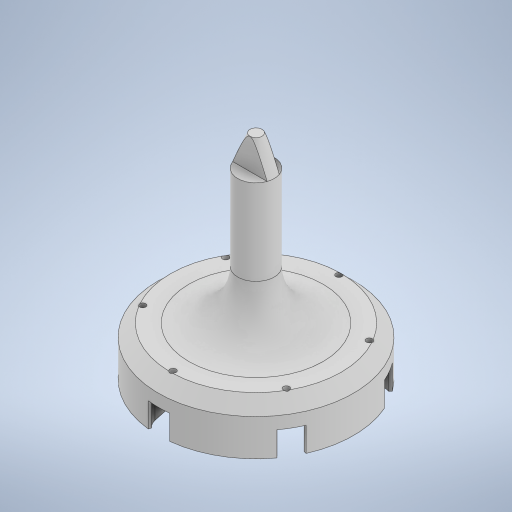
# Autodesk Inventor part: End_Effecto_simpler
Saved by Autodesk Inventor 2023 (Build 270158000, 158)
## iProperties
Created: 2025-02-16
Part Number: End_Effecto_simpler
Material: Generic
Document SubType Name: Modeling
Designer: Swoby
Density: 1 g/cm^3
Appearance: Default
Author: Swoby
Autodesk Inventor part; units mm, degrees
ref_plane "YZ Plane" through (0, 0, 0) normal (1, 0, 0) x (0, 1, 0)
ref_plane "XZ Plane" through (0, 0, 0) normal (0, 1, 0) x (-1, 0, 0)
ref_plane "XY Plane" through (0, 0, 0) normal (0, 0, 1) x (1, 0, 0)
sketch "Sketch1" plane through (0, 0, 0) normal (0, 0, 1) x (1, 0, 0)
  line L0 (0, 0) -> (0, 35)
  line L1 (0, 0) -> (-16, 0)
  line L2 (-16, 0) -> (-16, 8)
  line L3 (-3, 30) -> (0, 30) construction
  line L4 (-3, 30) -> (-3, 16)
  line L5 (-16, 8) -> (-11, 8)
  arc A0 (-11, 8) -> (-3, 16) centre (-11, 16) ccw
  line L6 (0, 35) -> (-1, 35)
  line L7 (-1, 35) -> (-3, 30)
  dimension "d0" = 32
  dimension "d1" = 30
  dimension "d2" = 6
  dimension "d4" = 8
  dimension "d7" = 8
  dimension "d8" = 5
  dimension "d10" = 1
  dimension "d34" = 8
  constraints: 16 end point, 3 horizontal, 2 point on circle, 2 vertical, 1 centre point, 1 parallel, 1 perpendicular, 1 point on line, 1 tangent
  measures "d0" diameter of L2 L0
  measures "d1" distance between parallel lines of L1 L3
  measures "d2" diameter of L3.start L0
  measures "d4" distance of L1.end L2.end
  measures "d7" distance from line of L5.end L4
  measures "d8" vertical distance of L3.start L0.end
  measures "d10" distance of L0.end L6.end
  measures "d34" distance from line of L4.end L5
revolve "Revolution1" add sketch "Sketch1" angle 360 about axis through (0, 0, 0) along (0, 1, 0)
chamfer "Chamfer1" distance 2 angle 45 1 edges at (16, 8, 0)
sketch "Sketch2" plane through (0, 0, 0) normal (0, -1, 0) x (1, 0, 0)
  arc A0 (-2.4436, -14.1282) -> (0, -16.1) centre (0, -13.6) ccw
  arc A1 (-13.943, -8.05) -> (-11.0136, -9.1803) centre (-11.7779, -6.8) ccw
  line L0 (0, -16.1) -> (0, 0) construction
  line L1 (0, 0) -> (-13.943, -8.05) construction
  circle A2 centre (0, 0) radius 8 construction
  line L2 (0, 0) -> (-4, -6.9282) construction
  line L3 (-3.9534, -7.1438) -> (-2.4436, -14.1282)
  line L4 (-4.21, -6.9956) -> (-11.0136, -9.1803)
  arc A3 (-3.9534, -7.1438) -> (-4.21, -6.9956) centre (-4.1489, -7.1861) ccw
  circle A4 centre (0, -13.6) radius 0.5
  circle A5 centre (11.7779, -6.8) radius 0.5
  arc A6 (11.0136, -9.1803) -> (13.943, -8.05) centre (11.7779, -6.8) ccw
  line L5 (4.21, -6.9956) -> (11.0136, -9.1803)
  arc A7 (4.21, -6.9956) -> (3.9534, -7.1438) centre (4.1489, -7.1861) ccw
  line L6 (3.9534, -7.1438) -> (2.4436, -14.1282)
  arc A8 (0, -16.1) -> (2.4436, -14.1282) centre (0, -13.6) ccw
  circle A9 centre (11.7779, 6.8) radius 0.5
  arc A10 (13.4572, 4.9479) -> (13.943, 8.05) centre (11.7779, 6.8) ccw
  line L7 (8.1634, 0.1482) -> (13.4572, 4.9479)
  arc A11 (8.1634, 0.1482) -> (8.1634, -0.1482) centre (8.2978, 0) ccw
  line L8 (8.1634, -0.1482) -> (13.4572, -4.9479)
  arc A12 (13.943, -8.05) -> (13.4572, -4.9479) centre (11.7779, -6.8) ccw
  circle A13 centre (0, 13.6) radius 0.5
  arc A14 (2.4436, 14.1282) -> (0, 16.1) centre (0, 13.6) ccw
  line L9 (3.9534, 7.1438) -> (2.4436, 14.1282)
  arc A15 (3.9534, 7.1438) -> (4.21, 6.9956) centre (4.1489, 7.1861) ccw
  line L10 (4.21, 6.9956) -> (11.0136, 9.1803)
  arc A16 (13.943, 8.05) -> (11.0136, 9.1803) centre (11.7779, 6.8) ccw
  circle A17 centre (-11.7779, 6.8) radius 0.5
  arc A18 (-11.0136, 9.1803) -> (-13.943, 8.05) centre (-11.7779, 6.8) ccw
  line L11 (-4.21, 6.9956) -> (-11.0136, 9.1803)
  arc A19 (-4.21, 6.9956) -> (-3.9534, 7.1438) centre (-4.1489, 7.1861) ccw
  line L12 (-3.9534, 7.1438) -> (-2.4436, 14.1282)
  arc A20 (0, 16.1) -> (-2.4436, 14.1282) centre (0, 13.6) ccw
  circle A21 centre (-11.7779, -6.8) radius 0.5
  arc A22 (-13.4572, -4.9479) -> (-13.943, -8.05) centre (-11.7779, -6.8) ccw
  line L13 (-8.1634, -0.1482) -> (-13.4572, -4.9479)
  arc A23 (-8.1634, -0.1482) -> (-8.1634, 0.1482) centre (-8.2978, 0) ccw
  line L14 (-8.1634, 0.1482) -> (-13.4572, 4.9479)
  arc A24 (-13.943, 8.05) -> (-13.4572, 4.9479) centre (-11.7779, 6.8) ccw
  point P0 (4, -6.9282)
  point P1 (8, 0)
  point P2 (4, 6.9282)
  point P3 (-4, 6.9282)
  point P4 (-8, 0)
  point P5 (0, -16.1)
  point P6 (0, 16.1)
  point P7 (-13.943, 8.05)
  dimension "d19" = 16
  dimension "d14" = 5
  dimension "d15" = 5
  dimension "d16" = 60
  dimension "d17" = 16.1
  dimension "d18" = 16.1
  dimension "d20" = 30
  dimension "d21" = 0.2
  dimension "d22" = 1
  dimension "d25" = 360
  constraints: 36 point on circle, 30 end point, 24 centre point, 14 point on line, 7 coincident, 4 tangent, 1 vertical, 106 other
  measures "d14" diameter of A0
  measures "d15" diameter of A1
  measures "d16" angle of L1 L0
  measures "d17" distance of L0.start L0.end
  measures "d18" distance of L0.end L1.end
  measures "d20" angle of L0 L2
  measures "d21" radius of A3
  measures "d22" diameter of A4
extrude "Extrusion1" cut sketch "Sketch2" against normal blind 4
extrude "Extrusion2" cut sketch "Sketch2" against normal through all contours A4 | A5 | A9 | A13 | A17 | A21
chamfer "Chamfer2" distance 1 angle 45 12 edges at (-13.4613, 2, -8.6483) (-14.2203, 2, -7.3336) (-14.2203, 2, 7.3336) (-13.4613, 2, 8.6483) (0.759, 2, 15.982) (14.2203, 2, 7.3336) (13.4613, 2, 8.6483) (14.2203, 2, -7.3336) (13.4613, 2, -8.6483) (0.759, 2, -15.982) (-0.759, 2, -15.982) (-0.759, 2, 15.982)
sketch "Sketch3" plane through (0, 35, 0) normal (0, 1, 0) x (1, 0, 0)
  circle A0 centre (0, 0) radius 1 projected
  circle A1 centre (0, 0) radius 3 projected
  line L0 (-2.8284, 1) -> (2.8284, 1)
  line L1 (-2.8284, -1) -> (2.8284, -1)
  constraints: 4 end point, 4 point on circle, 2 tangent, 1 horizontal, 1 parallel
extrude "Extrusion3" cut sketch "Sketch3" against normal blind 5 contours L0 A1 | L1 A1
equation "\"d7\" = d5"
equation "\"d18\" = d17"
equation "\"d20\" = 0.5 * d16"
equation "\"d5\" = 8"
body "Solid1"
